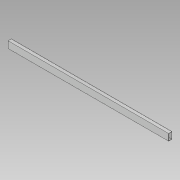
# Autodesk Inventor part: ALUMINUM
Saved by Autodesk Inventor 2020.1 (Build 241239000, 239)
## iProperties
Category: FIRST 2020 KOP
Company: Autodesk Inc.
Created: 2019-12-11
Part Number: ALUMINUM
Material: Aluminum 6061
Document SubType Name: Modeling
Designer: Autodesk Inc.
Density: 2.7 g/cm^3
Appearance: Aluminum - Polished
Catalog Web Link: https://www.hydro.com/Document/Index?name=Alloy%206063&id=5964
Vendor: Hydro Extrusion North America
Author: Autodesk Inc.
Autodesk Inventor part; units mm, degrees
ref_plane "YZ Plane" through (0, 0, 0) normal (1, 0, 0) x (0, 1, 0)
ref_plane "XZ Plane" through (0, 0, 0) normal (0, 1, 0) x (-1, 0, 0)
ref_plane "XY Plane" through (0, 0, 0) normal (0, 0, 1) x (1, 0, 0)
sketch "Sketch1" plane through (0, 0, 0) normal (0, 1, 0) x (-1, 0, 0)
  line L0 (0, 0) -> (25.4, 0)
  line L1 (25.4, 0) -> (25.4, -50.8)
  line L2 (25.4, -50.8) -> (0, -50.8)
  line L3 (0, -50.8) -> (0, 0)
  line L4 (23.8125, -49.2125) -> (23.8125, -1.5875)
  line L5 (23.8125, -1.5875) -> (1.5875, -1.5875)
  line L6 (1.5875, -1.5875) -> (1.5875, -49.2125)
  line L7 (1.5875, -49.2125) -> (23.8125, -49.2125)
  dimension "d0" = 25.4
  dimension "d1" = 50.8
  dimension "d2" = 1.5875
  constraints: 16 end point, 4 parallel, 2 perpendicular, 1 horizontal, 3 other
  measures "d0" distance of L1.end L2.end
  measures "d1" distance of L0.end L1.end
  measures "d2" distance between parallel lines of L1 L4
extrude "Extrusion1" add sketch "Sketch1" against normal blind 1219.2
body "Solid1"
